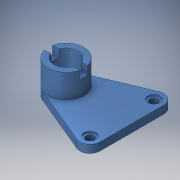
# Autodesk Inventor part: Workshop_1_Soln
Saved by Autodesk Inventor 2016 (Build 200138000, 138)
## iProperties
Created: 2017-07-15
Part Number: Workshop_1_Soln
Material: Bronze, Soft Tin
Document SubType Name: Modeling
Designer: bobbyl
Mass: 807.362 g
Surface Area: 253.061 cm^2
Volume: 90.9807 cm^3
Density: 8.874 g/cm^3
Appearance: Flaked Satin - Blue
Author: bobbyl
Autodesk Inventor part; units mm, degrees
ref_plane "YZ Plane" through (0, 0, 0) normal (1, 0, 0) x (0, 1, 0)
ref_plane "XZ Plane" through (0, 0, 0) normal (0, 1, 0) x (-1, 0, 0)
ref_plane "XY Plane" through (0, 0, 0) normal (0, 0, 1) x (1, 0, 0)
sketch "Sketch1" plane through (0, 0, 0) normal (0, 1, 0) x (-1, 0, 0)
  arc A0 (36.9231, -20.7692) -> (36.9231, 20.7692) centre (28.2692, 0) ccw
  line L0 (36.9231, 20.7692) -> (-36.9231, 51.5385)
  line L1 (36.9231, -20.7692) -> (-36.9231, -51.5385)
  arc A1 (-36.9231, 51.5385) -> (-54.2308, 40) centre (-41.7308, 40) ccw
  arc A2 (-54.2308, -40) -> (-36.9231, -51.5385) centre (-41.7308, -40) ccw
  line L2 (72.3868, 0) -> (-78.9359, 0) projected
  line L3 (0, -78.6378) -> (0, 78.6378) projected
  line L4 (-54.2308, 40) -> (-54.2308, -40)
  point P0 (0, 0)
  point P1 (0, -36.1538)
  point P2 (0, 36.1538)
  point P3 (-54.2308, 0)
  dimension "d0" = 70
  dimension "d1" = 80
  dimension "d2" = 12.5
  dimension "d3" = 45
  constraints: 6 end point, 6 point on circle, 6 tangent, 4 point on line, 3 centre point, 3 midpoint, 1 equal radius, 1 vertical
  measures "d0" horizontal distance of A1.centre A0.centre
  measures "d1" distance of A2.centre A1.centre
  measures "d2" radius of A1
  measures "d3" diameter of A0
extrude "Extrusion1" add sketch "Sketch1" along normal blind 10
sketch "Sketch2" plane through (0, 10, 0) normal (0, 1, 0) x (1, 0, 0)
  line L0 (-36.9231, -20.7692) -> (36.9231, -51.5385) projected
  arc A0 (36.9231, -51.5385) -> (54.2308, -40) centre (41.7308, -40) ccw projected
  line L1 (54.2308, -40) -> (54.2308, 40) projected
  arc A1 (54.2308, 40) -> (36.9231, 51.5385) centre (41.7308, 40) ccw projected
  line L2 (36.9231, 51.5385) -> (-36.9231, 20.7692) projected
  arc A2 (-36.9231, 20.7692) -> (-36.9231, -20.7692) centre (-28.2692, 0) ccw projected
  circle A3 centre (-28.2692, 0) radius 22.5
  point P0 (0, 0)
  constraints: 1 centre point, 1 coincident, 1 concentric
extrude "Extrusion2" add sketch "Sketch2" along normal blind 30 contours A2 A3
sketch "Sketch3" plane through (-28.2692, 40, 0) normal (0, 1, 0) x (1, 0, 0)
  circle A0 centre (0, 0) radius 15
  point P0 (28.2692, 0)
  dimension "d8" = 30
  constraints: 1 centre point
  measures "d8" diameter of A0
extrude "Extrusion3" cut sketch "Sketch3" against normal through all
sketch "Sketch4" plane through (-28.2692, 40, 0) normal (0, 1, 0) x (1, 0, 0)
  line L0 (-24.7308, -5) -> (25.2692, -5)
  line L1 (25.2692, -5) -> (25.2692, 5)
  line L2 (25.2692, 5) -> (-24.7308, 5)
  line L3 (-24.7308, 5) -> (-24.7308, -5)
  line L4 (-59.7, 0) -> (106.2, 0) projected
  line L5 (28.2692, 73.5) -> (28.2692, -73.5) projected
  point P0 (28.2692, 0)
  point P1 (-24.7308, 0)
  dimension "d14" = 10
  dimension "d15" = 50
  dimension "d16" = 3
  constraints: 8 end point, 2 parallel, 1 horizontal, 1 midpoint, 1 perpendicular, 1 point on line
  measures "d14" distance of L2.end L0.start
  measures "d15" distance of L1.end L2.end
  measures "d16" distance between parallel lines of L5 L1
extrude "Extrusion4" cut sketch "Sketch4" against normal blind 10
hole "Hole1" at (41.7308, 10, 40) direction (0, -1, 0) diameter 10 end through all counterbore diameter 15 counterbore depth 2
mirror "Mirror1" about plane through (0, 0, 0) normal (0, 0, 1) of "Hole1"
body "Solid1"
